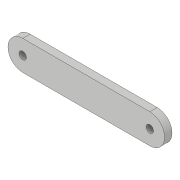
# Autodesk Inventor part: ScissorHookBar
Saved by Autodesk Inventor 2018 (Build 220112000, 112)
## iProperties
Created: 2020-01-27
Part Number: ScissorHookBar
Material: Generic
Document SubType Name: Modeling
Designer: Myers
Mass: 20.4315 g
Surface Area: 85.8227 cm^2
Volume: 20.4315 cm^3
Density: 1 g/cm^3
Appearance: Default
Author: Myers
Autodesk Inventor part; units mm, degrees
ref_plane "YZ Plane" through (0, 0, 0) normal (1, 0, 0) x (0, 1, 0)
ref_plane "XZ Plane" through (0, 0, 0) normal (0, 1, 0) x (-1, 0, 0)
ref_plane "XY Plane" through (0, 0, 0) normal (0, 0, 1) x (1, 0, 0)
sketch "Sketch1" plane through (0, 0, 0) normal (0, 0, 1) x (1, 0, 0)
  line L0 (0, 0) -> (109.22, 0) construction
  line L1 (0, -12.7) -> (109.22, -12.7)
  line L2 (109.22, 12.7) -> (0, 12.7)
  arc A0 (0, 12.7) -> (0, -12.7) centre (0, 0) ccw
  arc A1 (109.22, -12.7) -> (109.22, 12.7) centre (109.22, 0) ccw
  circle A2 centre (0, 0) radius 3.175
  circle A3 centre (109.22, 0) radius 3.175
  point P0 (54.61, 0)
  dimension "d0" = 25.4
  dimension "d1" = 109.22
  dimension "d2" = 6.35
  constraints: 8 end point, 4 centre point, 4 point on circle, 4 tangent, 2 coincident, 1 equal radius, 1 horizontal, 1 midpoint, 1 parallel
  measures "d0" diameter of A0
  measures "d1" distance of L0.start L0.end
  measures "d2" diameter of A2
extrude "Extrusion1" add sketch "Sketch1" along normal blind 6.35
body "Solid1"
